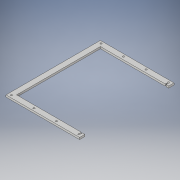
# Autodesk Inventor part: Top stabiliser
Saved by Autodesk Inventor 2019 (Build 230136000, 136)
## iProperties
Created: 2019-02-27
Part Number: Top stabiliser
Material: Generic
Document SubType Name: Modeling
Designer: aonih
Density: 1 g/cm^3
Appearance: Default
Author: aonih
Autodesk Inventor part; units mm, degrees
ref_plane "YZ Plane" through (0, 0, 0) normal (1, 0, 0) x (0, 1, 0)
ref_plane "XZ Plane" through (0, 0, 0) normal (0, 1, 0) x (-1, 0, 0)
ref_plane "XY Plane" through (0, 0, 0) normal (0, 0, 1) x (1, 0, 0)
sketch "Sketch2" plane through (0, 0, 0) normal (0, 1, 0) x (-1, 0, 0)
  line L0 (0, 195.5) -> (-22, 195.5)
  line L1 (-22, -195.5) -> (0, -195.5)
  line L2 (0, -195.5) -> (0, 195.5)
  line L3 (-22, 195.5) -> (-305, 195.5)
  line L4 (-305, 195.5) -> (-305, 173.5)
  line L5 (-305, 173.5) -> (-22, 173.5)
  line L6 (-22, -195.5) -> (-305, -195.5)
  line L7 (-305, -195.5) -> (-305, -173.5)
  line L8 (-305, -173.5) -> (-22, -173.5)
  circle A0 centre (-292.3, 185.5) radius 3.5
  line L9 (-292.3, 185.5) -> (-292.3, 173.5) construction
  line L10 (-289.7, 179.5) -> (-294.9, 179.5)
  line L11 (-294.9, 179.5) -> (-294.9, 173.5)
  line L12 (-294.9, 173.5) -> (-289.7, 173.5)
  line L13 (-289.7, 173.5) -> (-289.7, 179.5)
  circle A1 centre (-199.1, 185.5) radius 3.5
  circle A2 centre (-105.9, 185.5) radius 3.5
  circle A3 centre (-12.7, 185.5) radius 3.5
  line L14 (-22, 195.5) -> (-22, 173.5) construction
  line L15 (0, 0) -> (337.7885, 0) construction
  line L16 (0, 0) -> (-365.548, 0) construction
  line L17 (-22, 173.5) -> (-22, 0)
  line L18 (-22, -173.5) -> (-22, 0)
  circle A4 centre (-292.3, -185.5) radius 3.5
  line L19 (-289.7, -179.5) -> (-294.9, -179.5)
  line L20 (-294.9, -179.5) -> (-294.9, -173.5)
  line L21 (-289.7, -173.5) -> (-289.7, -179.5)
  circle A5 centre (-199.1, -185.5) radius 3.5
  circle A6 centre (-105.9, -185.5) radius 3.5
  circle A7 centre (-12.7, -185.5) radius 3.5
  line L22 (-294.9, -173.5) -> (-289.7, -173.5)
  dimension "d0" = 22
  dimension "d1" = 22
  dimension "d2" = 22
  dimension "d6" = 347
  dimension "d7" = 7
  dimension "d9" = 12.7
  dimension "d10" = 10
  dimension "d11" = 5.2
  dimension "d12" = 6
  dimension "d15" = 93.2
  dimension "d22" = 185.5
  dimension "d23" = 22
  dimension "d24" = 305
  dimension "d29" = 305
  constraints: 46 end point, 8 centre point, 8 symmetric about line, 7 horizontal, 5 parallel, 5 perpendicular, 2 collinear, 2 midpoint, 2 point on line, 1 coincident, 1 vertical, 10 other
  measures "d0" distance of L1.start L1.end
  measures "d1" distance of L6.end L7.end
  measures "d2" distance of L3.end L4.end
  measures "d6" distance between parallel lines of L8 L5
  measures "d7" diameter of A0
  measures "d9" distance from line of L4 L9.start
  measures "d10" distance from line of L3 L9.start
  measures "d11" distance of L12.end L11.end
  measures "d12" distance of L11.end L10.end
  measures "d15" distance of L9.start A1.centre
  measures "d22" distance from line of L16 A3.centre
  measures "d23" distance between parallel lines of L2 L17
  measures "d24" distance between parallel lines of L2 L4
  measures "d29" distance between parallel lines of L2 L7
extrude "Extrusion2" add sketch "Sketch2" along normal blind 8 contours L2 L1 L6 L7 L8 L20 L19 L21 L18 L17 L5 L13 L10 L11 L4 L3 L0
equation "\"d1\" = d0"
equation "\"d2\" = d0"
equation "\"d15\" = -0.666667 * d9 + 0.333333 * d24"
equation "\"d23\" = d0"
equation "\"d29\" = d24"
body "Solid2"
